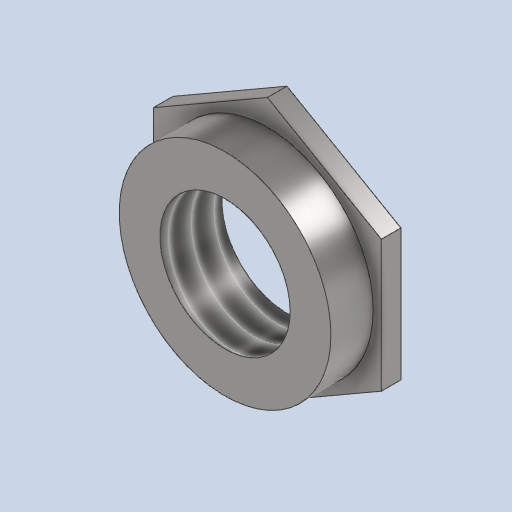
# Autodesk Inventor part: SF419
Saved by Autodesk Inventor 2022 (Build 260153000, 153)
## iProperties
Part Number: SF419
Material: チタン
Document SubType Name: Modeling
Designer: Masato Kubotera
Density: 6.98745 g/cm^3
Appearance: 半つや出し
Catalog Web Link: https://jp.misumi-ec.com/vona2/detail/221000555673/?HissuCode=SF419
Description: ReadyMade
Mass: 0.3125 g
Surface Area: 1.2471 cm^2
Volume: 0.044723 cm^3
Author: Masato Kubotera
Autodesk Inventor part; units mm, degrees
ref_plane "YZ Plane" through (0, 0, 0) normal (1, 0, 0) x (0, 1, 0)
ref_plane "XZ Plane" through (0, 0, 0) normal (0, 1, 0) x (-1, 0, 0)
ref_plane "XY Plane" through (0, 0, 0) normal (0, 0, 1) x (1, 0, 0)
sketch "スケッチ1" plane through (0, 0, 0) normal (0, 0, 1) x (1, 0, 0)
  circle A0 centre (0, 0) radius 3.25
  circle A1 centre (0, 0) radius 2
  line L0 (0, -4.0415) -> (-3.5, -2.0207)
  line L1 (-3.5, -2.0207) -> (-3.5, 2.0207)
  line L2 (-3.5, 2.0207) -> (0, 4.0415)
  line L3 (0, 4.0415) -> (3.5, 2.0207)
  line L4 (3.5, 2.0207) -> (3.5, -2.0207)
  line L5 (3.5, -2.0207) -> (0, -4.0415)
  dimension "d0" = 6.5
  dimension "d1" = 4
  dimension "d2" = 7
  constraints: 12 end point, 3 coincident, 2 centre point, 1 vertical, 13 other
  measures "d0" diameter of A0
  measures "d1" diameter of A1
  measures "d2" distance of L1.end L3.end
extrude "押し出し1" add sketch "スケッチ1" along normal blind 1.9 contours A0
extrude "押し出し2" add sketch "スケッチ1" along normal blind 0.6 contours L0 L1 L2 L3 L4 L5
thread "ねじ1" size "M4x0.7" class "6H" standard "ANSI Metric M Profile" full length
